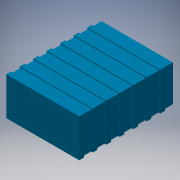
# Autodesk Inventor part: L16-TSV-8.1
Saved by Autodesk Inventor 2019 (Build 230136000, 136)
## iProperties
Created: 2013-02-18
Part Number: L16-TSV-8.1
Material: Generic
Document SubType Name: Modeling
Designer: user
Density: 1 g/cm^3
Mass: 1240.2 g
Surface Area: 825.366 cm^2
Volume: 1240.2 cm^3
Appearance: Sky Blue Medium
Description: BatteryBody
Author: user
Revision Number: 1
Autodesk Inventor part; units mm, degrees
ref_plane "YZ Plane" through (0, 0, 0) normal (1, 0, 0) x (0, 1, 0)
ref_plane "XZ Plane" through (0, 0, 0) normal (0, 1, 0) x (-1, 0, 0)
ref_plane "XY Plane" through (0, 0, 0) normal (0, 0, 1) x (1, 0, 0)
sketch "Sketch1" plane through (0, 0, 0) normal (0, 1, 0) x (-1, 0, 0)
  line L0 (62.25, -32.4) -> (-62.25, -32.4)
  line L1 (-62.25, -32.4) -> (-62.25, 32.4)
  line L2 (-62.25, 32.4) -> (62.25, 32.4)
  line L3 (62.25, 32.4) -> (62.25, -32.4)
  point P0 (0, 0)
  point P1 (62.25, 0)
  point P2 (0, -32.4)
  dimension "d0" = 124.5
  dimension "d2" = 64.8
  constraints: 8 end point, 2 midpoint, 2 parallel, 1 horizontal, 1 horizontal alignment, 1 perpendicular, 1 vertical alignment
  measures "d0" distance between parallel lines of L1 L3
  measures "d2" distance between parallel lines of L2 L0
extrude "Extrusion1" add sketch "Sketch1" along normal blind 161
sketch "Sketch2" plane through (-62.25, 0, 32.4) normal (0, 0, 1) x (1, 0, 0)
  line L0 (124.5, 0) -> (0, 0) projected
  line L1 (124.5, 0) -> (124.5, 161) projected
  line L2 (0, 0) -> (0, 161) projected
  line L3 (0, 23) -> (124.5, 23)
  line L4 (124.5, 23) -> (124.5, 8)
  line L5 (124.5, 8) -> (0, 8)
  line L6 (0, 8) -> (0, 23)
  line L7 (0, 31) -> (124.5, 31)
  line L8 (124.5, 31) -> (124.5, 46)
  line L9 (124.5, 46) -> (0, 46)
  line L10 (0, 46) -> (0, 31)
  line L11 (0, 54) -> (124.5, 54)
  line L12 (124.5, 54) -> (124.5, 69)
  line L13 (124.5, 69) -> (0, 69)
  line L14 (0, 69) -> (0, 54)
  line L15 (0, 77) -> (124.5, 77)
  line L16 (124.5, 77) -> (124.5, 92)
  line L17 (124.5, 92) -> (0, 92)
  line L18 (0, 92) -> (0, 77)
  line L19 (0, 100) -> (124.5, 100)
  line L20 (124.5, 100) -> (124.5, 115)
  line L21 (124.5, 115) -> (0, 115)
  line L22 (0, 115) -> (0, 100)
  line L23 (0, 123) -> (124.5, 123)
  line L24 (124.5, 123) -> (124.5, 138)
  line L25 (124.5, 138) -> (0, 138)
  line L26 (0, 138) -> (0, 123)
  line L27 (124.5, 146) -> (0, 146)
  line L28 (0, 146) -> (0, 161)
  line L29 (0, 161) -> (124.5, 161)
  line L30 (124.5, 161) -> (124.5, 146)
  point P0 (62.25, 0)
  dimension "d5" = 8
  dimension "d6" = 15
  dimension "d7" = 8
  dimension "d8" = 15
  dimension "d9" = 8
  dimension "d10" = 15
  dimension "d11" = 8
  dimension "d12" = 15
  dimension "d13" = 8
  dimension "d14" = 8
  dimension "d15" = 15
  dimension "d16" = 15
  dimension "d17" = 8
  dimension "d18" = 15
  constraints: 56 end point, 14 parallel, 7 horizontal, 7 perpendicular, 16 other
  measures "d5" distance between parallel lines of L0 L5
  measures "d6" distance between parallel lines of L5 L3
  measures "d7" distance between parallel lines of L3 L7
  measures "d8" distance between parallel lines of L7 L9
  measures "d9" distance between parallel lines of L9 L11
  measures "d10" distance between parallel lines of L11 L13
  measures "d11" distance between parallel lines of L13 L15
  measures "d12" distance between parallel lines of L15 L17
  measures "d13" distance between parallel lines of L17 L19
  measures "d14" distance between parallel lines of L23 L21
  measures "d15" distance between parallel lines of L19 L21
  measures "d16" distance between parallel lines of L23 L25
  measures "d17" distance between parallel lines of L25 L27
  measures "d18" distance between parallel lines of L27 L29
sketch "Sketch3" plane through (62.25, 0, -32.4) normal (0, 0, -1) x (-1, 0, 0)
  line L0 (0, 161) -> (124.5, 161) projected
  line L1 (0, 23) -> (124.5, 23)
  line L2 (124.5, 23) -> (124.5, 8)
  line L3 (124.5, 8) -> (0, 8)
  line L4 (0, 8) -> (0, 23)
  line L5 (0, 31) -> (124.5, 31)
  line L6 (124.5, 31) -> (124.5, 46)
  line L7 (124.5, 46) -> (0, 46)
  line L8 (0, 46) -> (0, 31)
  line L9 (0, 54) -> (124.5, 54)
  line L10 (124.5, 54) -> (124.5, 69)
  line L11 (124.5, 69) -> (0, 69)
  line L12 (0, 69) -> (0, 54)
  line L13 (0, 77) -> (124.5, 77)
  line L14 (124.5, 77) -> (124.5, 92)
  line L15 (124.5, 92) -> (0, 92)
  line L16 (0, 92) -> (0, 77)
  line L17 (0, 100) -> (124.5, 100)
  line L18 (124.5, 100) -> (124.5, 115)
  line L19 (124.5, 115) -> (0, 115)
  line L20 (0, 115) -> (0, 100)
  line L21 (0, 123) -> (124.5, 123)
  line L22 (124.5, 123) -> (124.5, 138)
  line L23 (124.5, 138) -> (0, 138)
  line L24 (0, 138) -> (0, 123)
  line L25 (124.5, 146) -> (0, 146)
  line L26 (0, 146) -> (0, 161)
  line L27 (0, 161) -> (124.5, 161)
  line L28 (124.5, 161) -> (124.5, 146)
  point P0 (62.25, 0)
  point P1 (62.25, 0)
  dimension "d20" = 15
  dimension "d21" = 8
  dimension "d22" = 15
  dimension "d23" = 8
  dimension "d24" = 15
  dimension "d25" = 8
  dimension "d26" = 15
  dimension "d27" = 8
  dimension "d28" = 8
  dimension "d29" = 15
  dimension "d30" = 15
  dimension "d31" = 8
  dimension "d32" = 15
  constraints: 56 end point, 14 parallel, 7 horizontal, 7 perpendicular, 1 collinear
  measures "d20" distance between parallel lines of L3 L1
  measures "d21" distance between parallel lines of L1 L5
  measures "d22" distance between parallel lines of L5 L7
  measures "d23" distance between parallel lines of L7 L9
  measures "d24" distance between parallel lines of L9 L11
  measures "d25" distance between parallel lines of L11 L13
  measures "d26" distance between parallel lines of L13 L15
  measures "d27" distance between parallel lines of L15 L17
  measures "d28" distance between parallel lines of L21 L19
  measures "d29" distance between parallel lines of L17 L19
  measures "d30" distance between parallel lines of L21 L23
  measures "d31" distance between parallel lines of L23 L25
  measures "d32" distance between parallel lines of L25 L27
extrude "Extrusion2" cut sketch "Sketch3" against normal blind 1.5
extrude "Extrusion3" cut sketch "Sketch2" against normal blind 1.5 contours L5 L2 L3 L1 | L7 L2 L9 L1 | L11 L2 L13 L1 | L15 L2 L17 L1 | L19 L2 L21 L1 | L23 L2 L25 L1 | L27 L2 L29 L1
sketch "Sketch5" plane through (62.25, 0, 32.4) normal (1, 0, 0) x (0, 0, -1)
  line L0 (1.5, 161) -> (63.3, 161)
  line L1 (63.3, 161) -> (63.3, 146)
  line L2 (63.3, 146) -> (1.5, 146)
  line L3 (1.5, 146) -> (1.5, 161)
  line L4 (1.5, 138) -> (63.3, 138)
  line L5 (63.3, 138) -> (63.3, 123)
  line L6 (63.3, 123) -> (1.5, 123)
  line L7 (1.5, 123) -> (1.5, 138)
  line L8 (1.5, 115) -> (63.3, 115)
  line L9 (63.3, 115) -> (63.3, 100)
  line L10 (63.3, 100) -> (1.5, 100)
  line L11 (1.5, 100) -> (1.5, 115)
  line L12 (1.5, 92) -> (63.3, 92)
  line L13 (63.3, 92) -> (63.3, 77)
  line L14 (63.3, 77) -> (1.5, 77)
  line L15 (1.5, 77) -> (1.5, 92)
  line L16 (1.5, 69) -> (63.3, 69)
  line L17 (63.3, 69) -> (63.3, 54)
  line L18 (63.3, 54) -> (1.5, 54)
  line L19 (1.5, 54) -> (1.5, 69)
  line L20 (1.5, 46) -> (63.3, 46)
  line L21 (63.3, 46) -> (63.3, 31)
  line L22 (63.3, 31) -> (1.5, 31)
  line L23 (1.5, 31) -> (1.5, 46)
  line L24 (1.5, 23) -> (63.3, 23)
  line L25 (63.3, 23) -> (63.3, 8)
  line L26 (63.3, 8) -> (1.5, 8)
  line L27 (1.5, 8) -> (1.5, 23)
  point P0 (32.4, 0)
  constraints: 56 end point, 14 parallel, 7 horizontal, 7 perpendicular
sketch "Sketch6" plane through (-62.25, 0, -32.4) normal (-1, 0, 0) x (0, 0, 1)
  line L0 (1.5, 161) -> (63.3, 161) projected
  line L1 (1.5, 161) -> (1.5, 146) projected
  line L2 (1.5, 161) -> (63.3, 161)
  line L3 (63.3, 161) -> (63.3, 146)
  line L4 (63.3, 146) -> (1.5, 146)
  line L5 (1.5, 146) -> (1.5, 161)
  line L6 (63.3, 138) -> (1.5, 138)
  line L7 (1.5, 138) -> (1.5, 123)
  line L8 (1.5, 123) -> (63.3, 123)
  line L9 (63.3, 123) -> (63.3, 138)
  line L10 (1.5, 115) -> (63.3, 115)
  line L11 (63.3, 115) -> (63.3, 100)
  line L12 (63.3, 100) -> (1.5, 100)
  line L13 (1.5, 100) -> (1.5, 115)
  line L14 (1.5, 92) -> (63.3, 92)
  line L15 (63.3, 92) -> (63.3, 77)
  line L16 (63.3, 77) -> (1.5, 77)
  line L17 (1.5, 77) -> (1.5, 92)
  line L18 (63.3, 69) -> (1.5, 69)
  line L19 (1.5, 69) -> (1.5, 54)
  line L20 (1.5, 54) -> (63.3, 54)
  line L21 (63.3, 54) -> (63.3, 69)
  line L22 (1.5, 46) -> (63.3, 46)
  line L23 (63.3, 46) -> (63.3, 31)
  line L24 (63.3, 31) -> (1.5, 31)
  line L25 (1.5, 31) -> (1.5, 46)
  line L26 (63.3, 23) -> (1.5, 23)
  line L27 (1.5, 23) -> (1.5, 8)
  line L28 (1.5, 8) -> (63.3, 8)
  line L29 (63.3, 8) -> (63.3, 23)
  point P0 (32.4, 0)
  constraints: 56 end point, 14 parallel, 7 horizontal, 7 perpendicular, 1 collinear, 1 point on line
extrude "Extrusion4" cut sketch "Sketch6" against normal blind 1.5
extrude "Extrusion5" cut sketch "Sketch5" against normal blind 1.5
equation "\"d0\" = BtWd"
equation "\"d2\" = BtDp"
equation "\"d3\" = BatteryHt"
equation "\"d5\" = RidgeWd"
equation "\"d6\" = RidgeGapWd"
equation "\"d7\" = d5"
equation "\"d8\" = d6"
equation "\"d9\" = d7"
equation "\"d10\" = d6"
equation "\"d11\" = d5"
equation "\"d12\" = d6"
equation "\"d13\" = d5"
equation "\"d14\" = d5"
equation "\"d15\" = d6"
equation "\"d16\" = d15"
equation "\"d17\" = d14"
equation "\"d18\" = d16"
equation "\"d20\" = d34"
equation "\"d21\" = d19"
equation "\"d22\" = d20"
equation "\"d23\" = d21"
equation "\"d24\" = d20"
equation "\"d25\" = d19"
equation "\"d26\" = d20"
equation "\"d27\" = d19"
equation "\"d28\" = d19"
equation "\"d29\" = d20"
equation "\"d30\" = d29"
equation "\"d31\" = d28"
equation "\"d32\" = d30"
equation "\"d36\" = RidgeThickness"
equation "\"d38\" = RidgeThickness"
equation "\"d40\" = RidgeThickness"
equation "\"d42\" = RidgeThickness"
equation "\"d19\" = d33"
equation "\"BtWd\" = 124.5"
equation "\"BtDp\" = 64.8"
equation "\"BatteryHt\" = 161"
equation "\"RidgeWd\" = 8"
equation "\"RidgeGapWd\" = 15"
equation "\"d34\" = 15"
equation "\"RidgeThickness\" = 1.5"
equation "\"d33\" = 8"
body "Solid1"
